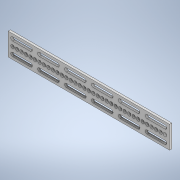
# Autodesk Inventor part: QuickPrototypeplateB
Saved by Autodesk Inventor 2020 (Build 240168000, 168)
## iProperties
Created: 2020-01-06
Part Number: QuickPrototypeplateB
Material: Generic
Document SubType Name: Modeling
Designer: srini
Density: 1 g/cm^3
Appearance: Default
Author: srini
Autodesk Inventor part; units mm, degrees
ref_plane "YZ Plane" through (0, 0, 0) normal (1, 0, 0) x (0, 1, 0)
ref_plane "XZ Plane" through (0, 0, 0) normal (0, 1, 0) x (-1, 0, 0)
ref_plane "XY Plane" through (0, 0, 0) normal (0, 0, 1) x (1, 0, 0)
sketch "Sketch1" plane through (0, 0, 0) normal (0, 0, 1) x (1, 0, 0)
  line L0 (-114.3, -15.875) -> (114.3, -15.875)
  line L1 (114.3, -15.875) -> (114.3, 15.875)
  line L2 (114.3, 15.875) -> (-114.3, 15.875)
  line L3 (-114.3, 15.875) -> (-114.3, -15.875)
  line L4 (-114.3, -15.875) -> (114.3, 15.875) construction
  line L5 (114.3, -15.875) -> (-114.3, 15.875) construction
  line L6 (-107.95, 9.525) -> (-82.55, 9.525) construction
  line L7 (-107.95, 6.9596) -> (-82.55, 6.9596)
  line L8 (-82.55, 12.0904) -> (-107.95, 12.0904)
  arc A0 (-107.95, 12.0904) -> (-107.95, 6.9596) centre (-107.95, 9.525) ccw
  arc A1 (-82.55, 6.9596) -> (-82.55, 12.0904) centre (-82.55, 9.525) ccw
  line L9 (-69.85, 9.525) -> (-44.45, 9.525) construction
  line L10 (-69.85, 6.9596) -> (-44.45, 6.9596)
  line L11 (-44.45, 12.0904) -> (-69.85, 12.0904)
  arc A2 (-69.85, 12.0904) -> (-69.85, 6.9596) centre (-69.85, 9.525) ccw
  arc A3 (-44.45, 6.9596) -> (-44.45, 12.0904) centre (-44.45, 9.525) ccw
  line L12 (-31.75, 9.525) -> (-6.35, 9.525) construction
  line L13 (-31.75, 6.9596) -> (-6.35, 6.9596)
  line L14 (-6.35, 12.0904) -> (-31.75, 12.0904)
  arc A4 (-31.75, 12.0904) -> (-31.75, 6.9596) centre (-31.75, 9.525) ccw
  arc A5 (-6.35, 6.9596) -> (-6.35, 12.0904) centre (-6.35, 9.525) ccw
  line L15 (6.35, 9.525) -> (31.75, 9.525) construction
  line L16 (6.35, 6.9596) -> (31.75, 6.9596)
  line L17 (31.75, 12.0904) -> (6.35, 12.0904)
  arc A6 (6.35, 12.0904) -> (6.35, 6.9596) centre (6.35, 9.525) ccw
  arc A7 (31.75, 6.9596) -> (31.75, 12.0904) centre (31.75, 9.525) ccw
  line L18 (44.45, 9.525) -> (69.85, 9.525) construction
  line L19 (44.45, 6.9596) -> (69.85, 6.9596)
  line L20 (69.85, 12.0904) -> (44.45, 12.0904)
  arc A8 (44.45, 12.0904) -> (44.45, 6.9596) centre (44.45, 9.525) ccw
  arc A9 (69.85, 6.9596) -> (69.85, 12.0904) centre (69.85, 9.525) ccw
  line L21 (82.55, 9.525) -> (107.95, 9.525) construction
  line L22 (82.55, 6.9596) -> (107.95, 6.9596)
  line L23 (107.95, 12.0904) -> (82.55, 12.0904)
  arc A10 (82.55, 12.0904) -> (82.55, 6.9596) centre (82.55, 9.525) ccw
  arc A11 (107.95, 6.9596) -> (107.95, 12.0904) centre (107.95, 9.525) ccw
  line L24 (-107.95, -9.525) -> (-82.55, -9.525) construction
  line L25 (-107.95, -12.0904) -> (-82.55, -12.0904)
  line L26 (-82.55, -6.9596) -> (-107.95, -6.9596)
  arc A12 (-107.95, -6.9596) -> (-107.95, -12.0904) centre (-107.95, -9.525) ccw
  arc A13 (-82.55, -12.0904) -> (-82.55, -6.9596) centre (-82.55, -9.525) ccw
  line L27 (-69.85, -9.525) -> (-44.45, -9.525) construction
  line L28 (-69.85, -12.0904) -> (-44.45, -12.0904)
  line L29 (-44.45, -6.9596) -> (-69.85, -6.9596)
  arc A14 (-69.85, -6.9596) -> (-69.85, -12.0904) centre (-69.85, -9.525) ccw
  arc A15 (-44.45, -12.0904) -> (-44.45, -6.9596) centre (-44.45, -9.525) ccw
  line L30 (-31.75, -9.525) -> (-6.35, -9.525) construction
  line L31 (-31.75, -12.0904) -> (-6.35, -12.0904)
  line L32 (-6.35, -6.9596) -> (-31.75, -6.9596)
  arc A16 (-31.75, -6.9596) -> (-31.75, -12.0904) centre (-31.75, -9.525) ccw
  arc A17 (-6.35, -12.0904) -> (-6.35, -6.9596) centre (-6.35, -9.525) ccw
  line L33 (6.35, -9.525) -> (31.75, -9.525) construction
  line L34 (6.35, -12.0904) -> (31.75, -12.0904)
  line L35 (31.75, -6.9596) -> (6.35, -6.9596)
  arc A18 (6.35, -6.9596) -> (6.35, -12.0904) centre (6.35, -9.525) ccw
  arc A19 (31.75, -12.0904) -> (31.75, -6.9596) centre (31.75, -9.525) ccw
  line L36 (44.45, -9.525) -> (69.85, -9.525) construction
  line L37 (44.45, -12.0904) -> (69.85, -12.0904)
  line L38 (69.85, -6.9596) -> (44.45, -6.9596)
  arc A20 (44.45, -6.9596) -> (44.45, -12.0904) centre (44.45, -9.525) ccw
  arc A21 (69.85, -12.0904) -> (69.85, -6.9596) centre (69.85, -9.525) ccw
  line L39 (82.55, -9.525) -> (107.95, -9.525) construction
  line L40 (82.55, -12.0904) -> (107.95, -12.0904)
  line L41 (107.95, -6.9596) -> (82.55, -6.9596)
  arc A22 (82.55, -6.9596) -> (82.55, -12.0904) centre (82.55, -9.525) ccw
  arc A23 (107.95, -12.0904) -> (107.95, -6.9596) centre (107.95, -9.525) ccw
  circle A24 centre (-107.95, 0) radius 2.4892
  circle A25 centre (-101.6, 0) radius 2.4892
  circle A26 centre (-95.25, 0) radius 2.4892
  circle A27 centre (-88.9, 0) radius 2.4892
  circle A28 centre (-82.55, 0) radius 2.4892
  circle A29 centre (-76.2, 0) radius 2.4892
  circle A30 centre (-69.85, 0) radius 2.4892
  circle A31 centre (-63.5, 0) radius 2.4892
  circle A32 centre (-57.15, 0) radius 2.4892
  circle A33 centre (-50.8, 0) radius 2.4892
  circle A34 centre (-44.45, 0) radius 2.4892
  circle A35 centre (-38.1, 0) radius 2.4892
  circle A36 centre (-31.75, 0) radius 2.4892
  circle A37 centre (-25.4, 0) radius 2.4892
  circle A38 centre (-19.05, 0) radius 2.4892
  circle A39 centre (-12.7, 0) radius 2.4892
  circle A40 centre (-6.35, 0) radius 2.4892
  circle A41 centre (0, 0) radius 2.4892
  circle A42 centre (6.35, 0) radius 2.4892
  circle A43 centre (12.7, 0) radius 2.4892
  circle A44 centre (19.05, 0) radius 2.4892
  circle A45 centre (25.4, 0) radius 2.4892
  circle A46 centre (31.75, 0) radius 2.4892
  circle A47 centre (38.1, 0) radius 2.4892
  circle A48 centre (44.45, 0) radius 2.4892
  circle A49 centre (50.8, 0) radius 2.4892
  circle A50 centre (57.15, 0) radius 2.4892
  circle A51 centre (63.5, 0) radius 2.4892
  circle A52 centre (69.85, 0) radius 2.4892
  circle A53 centre (76.2, 0) radius 2.4892
  circle A54 centre (82.55, 0) radius 2.4892
  circle A55 centre (88.9, 0) radius 2.4892
  circle A56 centre (95.25, 0) radius 2.4892
  circle A57 centre (101.6, 0) radius 2.4892
  circle A58 centre (107.95, 0) radius 2.4892
  point P0 (0, 0)
  point P1 (-95.25, 9.525)
  point P2 (-57.15, 9.525)
  point P3 (-19.05, 9.525)
  point P4 (19.05, 9.525)
  point P5 (57.15, 9.525)
  point P6 (95.25, 9.525)
  point P7 (-95.25, -9.525)
  point P8 (-57.15, -9.525)
  point P9 (-19.05, -9.525)
  point P10 (19.05, -9.525)
  point P11 (57.15, -9.525)
  point P12 (95.25, -9.525)
  dimension "d0" = 228.6
  dimension "d1" = 31.75
  dimension "d2" = 2.5654
  dimension "d3" = 25.4
  dimension "d4" = 6.35
  dimension "d5" = 6.35
  dimension "d8" = 38.1
  dimension "d11" = 19.05
  dimension "d14" = 6.35
  dimension "d17" = 6.35
  dimension "d22" = 4.9784
  constraints: 108 end point, 59 centre point, 48 point on circle, 4 horizontal, 4 tangent, 3 midpoint, 3 parallel, 1 perpendicular, 1 vertical, 200 other
  measures "d0" distance of L1.end L2.end
  measures "d1" distance of L2.end L0.start
  measures "d2" radius of A1
  measures "d3" distance of L6.start L6.end
  measures "d4" distance between parallel lines of L6 L2
  measures "d5" distance from line of L3 L6.start
  measures "d8" distance of L7.start L10.start
  measures "d11" distance of L7.start L25.start
  measures "d14" distance from line of L3 A24.centre
  measures "d17" distance of A24.centre A25.centre
  measures "d22" diameter of A24
extrude "Extrusion1" add sketch "Sketch1" along normal blind 3.175
body "Solid1"
